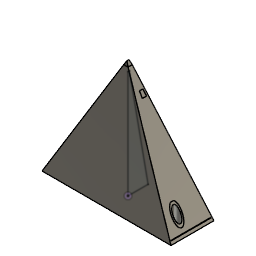
BoTech.StarClock.StarPeak (Autodesk Fusion 360 design; units mm, degrees)
Autodesk Fusion 360 part; units mm, degrees
note: some values were not read from the file. Set by a fixed rule: which sketch regions a step uses.
sketch "Skizze1" plane through (0, 0, 0) normal (0, 1, 0) x (1, 0, 0)
  line L0 (-45, -0.0577) -> (45, -0.0577)
  line L1 (0, -82.1154) -> (-45, -0.0577)
  line L2 (-45, -0.0577) -> (12.5, -0.0577)
  line L3 (45, -0.0577) -> (0, -82.1154)
  line L4 (-1.5, -79.3) -> (1.494, -79.3)
  line L5 (1.494, -79.3) -> (1.544, -79.3)
  line L6 (-1.5, -79.3) -> (-1.544, -79.3)
  dimension "d1" = 57.5
  dimension "d2" = 82.0577
  constraint parallel L0 L2
  constraint coincident L3 L5.end
  constraint parallel L4 L5
  constraint coincident L1 L6.end
  constraint parallel L4 L6
  measures "d1" distance of L0.start L2.end
  measures "d2" distance of L1.start L2
sketch "Skizze2" plane through (0, 0, 0) normal (0, 0, 1) x (1, 0, 0)
  line L0 (22, 10) -> (22, -10)
  line L1 (-45, -15) -> (45, -15)
  line L2 (45, -15) -> (45, 15)
  line L3 (-45, 15) -> (-45, -15)
  line L4 (39, 0) -> (39, -5)
  line L5 (22, -10) -> (-22, -10)
  line L6 (-22, 0) -> (-39, 0)
  line L7 (-45, 15) -> (45, 15)
  circle A0 centre (39, -5) radius 3.5
  circle A1 centre (-39, 5) radius 3.5
  line L8 (45, 0) -> (39, 0)
  circle A2 centre (39, -5) radius 2.5
  line L9 (39, 0) -> (22, 0)
  line L10 (-22, 10) -> (22, 10)
  line L11 (-39, 0) -> (-45, 0)
  arc A3 (22, -10) -> (22, 10) centre (22, 0) ccw
  line L12 (45, 15) -> (45, -15)
  arc A4 (-22, 10) -> (-22, -10) centre (-22, 0) ccw
  circle A5 centre (39, -5) radius 1
  line L13 (45, -15) -> (-45, -15)
  circle A6 centre (-39, 5) radius 2.5
  line L14 (-45, -15) -> (-45, 15)
  line L15 (-39, 0) -> (-39, 5)
  line L16 (22, 0) -> (-22, 0)
  circle A7 centre (-39, 5) radius 1
  line L17 (-45, 14) -> (-44, 14)
  line L18 (-44, 14) -> (44, 14)
  line L19 (44, 14) -> (44, -14)
  line L20 (44, -14) -> (-44, -14)
  line L21 (-44, -14) -> (-44, 14)
  line L22 (-34, 14) -> (-34, -14)
  line L23 (33.9998, 14) -> (33.9998, -14)
  line L24 (-44, -14) -> (-45, -14)
  line L25 (44, -14) -> (45, -14)
  line L26 (44, 14) -> (45, 14)
  point P0 (0, -15)
  point P1 (-39, 5)
  dimension "d3" = 2
  dimension "d4" = 5
  dimension "d5" = 6
  dimension "d6" = 17
  dimension "d7" = 44
  dimension "d8" = 17
  dimension "d9" = 6
  dimension "d10" = 2
  dimension "d11" = 5
  dimension "d12" = 5
  dimension "d13" = 5
  dimension "d14" = 1
  constraint perpendicular L0 L5
  constraint tangent L10 A4
  constraint tangent L5 A3
  constraint concentric A2 A5
  constraint concentric A0 A2
  constraint horizontal L7
  constraint vertical L12
  constraint horizontal L13
  constraint vertical L14
  constraint coincident L1.end L2.start
  constraint coincident L3.start L7.start
  constraint midpoint L8.start L12
  constraint perpendicular L8 L12
  constraint parallel L8 L9
  constraint perpendicular L0 L16
  constraint perpendicular L11 L14
  constraint concentric A6 A7
  constraint concentric A1 A6
  constraint coincident P1 A1.centre
  constraint perpendicular L6 L15
  constraint perpendicular L4 L8
  constraint coincident L4.end A0.centre
  constraint coincident L3 L17.start
  constraint perpendicular L3 L17
  constraint horizontal L18
  constraint vertical L19
  constraint horizontal L20
  constraint vertical L21
  constraint coincident L18 L22.start
  constraint coincident L20 L22.end
  constraint coincident L18 L23.start
  constraint coincident L20 L23.end
  constraint coincident L14 L24.end
  constraint perpendicular L14 L24
  constraint coincident L12 L25.end
  constraint perpendicular L12 L25
  constraint coincident L12 L26.end
  constraint perpendicular L12 L26
  measures "d3" diameter of A5
  measures "d4" diameter of A2
  measures "d5" distance of L8.start L4.start
  measures "d6" distance of L9.end L4.start
  measures "d7" distance of L9.end L6.start
  measures "d8" distance of L6.start L6.end
  measures "d9" distance of L6.end L11.end
  measures "d10" diameter of A7 origin
  measures "d11" diameter of A6 origin
  measures "d12" distance of L6.end P1
  measures "d13" distance of L4.start L4.end
  measures "d14" distance of L17.start L17.end
ref_plane "Arbeitsebene1" through (0, 0, 79.3) normal (0, 0, 1) x (1, 0, 0)
sketch "Skizze4" plane through (0, 0, 79.3) normal (0, 0, 1) x (1, 0, 0)
  line L0 (-1.5, 1.5) -> (1.5, 1.5)
  line L1 (1.5, 1.5) -> (1.5, -1.5)
  line L2 (1.5, -1.5) -> (-1.5, -1.5)
  line L3 (-1.5, -1.5) -> (-1.5, 1.5)
  line L4 (-1.5, -0.5) -> (1.5, -0.5)
  line L5 (1.5, 0.5) -> (-1.5, 0.5)
  line L6 (0.5, 0.5) -> (0.5, -0.5)
  line L7 (-0.5, -0.5) -> (-0.5, 0.5)
  dimension "d17" = 3
  dimension "d18" = 3
  constraint horizontal L0
  constraint vertical L1
  constraint horizontal L2
  constraint vertical L3
  constraint coincident L3 L4.start
  constraint coincident L1 L4.end
  constraint perpendicular L1 L4
  constraint coincident L1 L5.start
  constraint coincident L3 L5.end
  constraint perpendicular L3 L5
  constraint coincident L5 L6.start
  constraint perpendicular L5 L6
  constraint coincident L4 L7.start
  constraint coincident L5 L7.end
  constraint perpendicular L5 L7
  measures "d17" distance of L0.start L0.end
  measures "d18" distance of L0.start L2.end
loft "Erhebung1" add profiles "Skizze2", "Skizze4" section 1 contours L1 L2 L3 L12 L13 L14 L20 L24 L25 section 2 contours L1 L2 L3 L4
loft "Erhebung2" add profiles "Skizze2", "Skizze4" section 1 contours L2 L8 L12 L19 L26 | L2 L8 L12 L19 L25 section 2 contours L1 L4 L5 L6
loft "Erhebung3" add profiles "Skizze2", "Skizze4" section 1 contours L2 L3 L7 L12 L14 L17 L18 L26 section 2 contours L0 L1 L3 L5
loft "Erhebung4" add profiles "Skizze2", "Skizze4" section 1 contours L3 L11 L14 L21 L24 | L3 L11 L14 L17 L21 section 2 contours L3 L4 L5 L7
sketch "Skizze5" plane through (0, 0, 0) normal (0, 1, 0) x (1, 0, 0)
  line L0 (-1.5, -79.3) -> (1.5, -79.3)
  line L1 (1.5, -79.3) -> (0, -82)
  line L2 (0, -82) -> (-1.5, -79.3)
  constraint horizontal L0
extrude "Extrusion2" add sketch "Skizze5" along normal blind -1.5 and the other way blind -1.5
sketch "Skizze6" plane through (0, 0, 0) normal (1, 0, 0) x (0, 1, 0)
  line L0 (1.5, 79.3) -> (0.7, 82)
  line L1 (-1.5, 79.3) -> (-0.7, 82)
  line L2 (-0.7, 82) -> (0.7, 82)
  line L3 (1.5, 79.3) -> (-1.5, 79.3)
  line L4 (1.5, 79.3) -> (1.5, 82)
  line L5 (1.5, 82) -> (0.7, 82)
  line L6 (-0.7, 82) -> (-1.5, 82)
  line L7 (-1.5, 82) -> (-1.5, 79.3)
  constraint horizontal L2
  constraint parallel L2 L3
  constraint perpendicular L3 L4
  constraint perpendicular L4 L5
  constraint parallel L2 L6
  constraint perpendicular L3 L7
extrude "Extrusion3" cut sketch "Skizze6" along normal blind 1.5 and the other way blind 1.5 contours L0 L4 L5 | L1 L6 L7
extrude "Extrusion4" add sketch "Skizze2" along normal blind 2 contours L8 L9 L18 L19 L23 | L8 L9 L19 L20 L23 | L6 L11 L20 L21 L22 | L6 L11 L18 L21 L22 | A0 | A1 | A2 | A6
extrude "Extrusion5" cut sketch "Skizze2" along normal blind 15 from surface at 2 contours A2 | A5 | A6 | A7
extrude "Extrusion6" add sketch "Skizze2" along normal blind 17 contours A0 | A1
sketch "Skizze8" plane through (0, 0, 0) normal (1, 0, 0) x (0, 1, 0)
  line L0 (0, 75) -> (0, 0)
  line L1 (0, 0) -> (14, 0)
  line L2 (0, 75) -> (1, 75)
  line L3 (1, 75) -> (14, 0)
  dimension "d43" = 14
  dimension "d44" = 75
  dimension "d45" = 1
  constraint coincident L0.end L1.start
  constraint vertical L0
  constraint perpendicular L0 L1
  constraint perpendicular L0 L2
  measures "d43" distance of L0.end L1.end
  measures "d44" distance of L0.start L0.end
  measures "d45" distance of L0.start L2.end
extrude "Extrusion8" add sketch "Skizze8" along normal blind 2 from surface at 8
extrude "Extrusion9" add sketch "Skizze8" along normal blind 2 from surface at -8.25
sketch "Skizze7" plane through (0, 0, 0) normal (0, 1, 0) x (1, 0, 0)
  line L0 (-45, 0) -> (-1.5, -79.3)
  line L1 (-45, 0) -> (-45, -79.3)
  line L2 (-45, -79.3) -> (-1.5, -79.3)
  line L3 (0, 0) -> (0, -1)
  line L4 (0, -1) -> (0, -12)
  line L5 (45, 0) -> (1.5, -79.3)
  line L6 (45, -79.3) -> (1.5, -79.3)
  line L7 (45, 0) -> (45, -79.3)
  constraint vertical L1
  constraint coincident L3.start origin
  constraint vertical L3
  constraint parallel L3 L4
  constraint symmetric L0.start L4 L5.start
  constraint symmetric L0.end L4 L5.end
  constraint symmetric L1.end L4 L6.start
extrude "Extrusion7" cut sketch "Skizze7" along normal blind 15 and the other way blind 15
